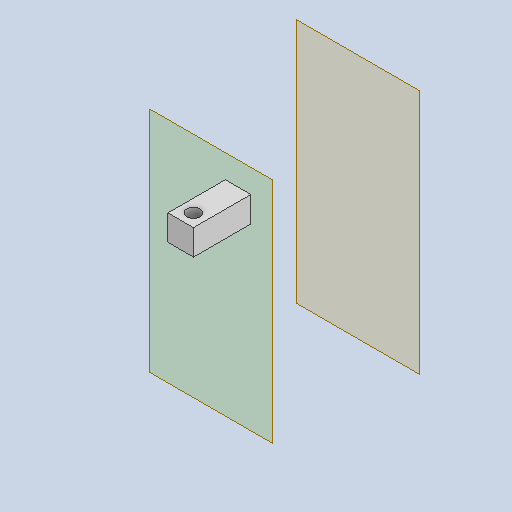
# Autodesk Inventor part: Refuerzo superior
Saved by Autodesk Inventor 2024 (Build 280153000, 153)
## iProperties
Created: 2025-03-01
Part Number: Refuerzo superior
Material: Genérico
Document SubType Name: Modeling
Designer: sergi
Density: 1 g/cm^3
Appearance: Valor por defecto
Author: sergi
Autodesk Inventor part; units mm, degrees
ref_plane "YZ Plane" through (0, 0, 0) normal (1, 0, 0) x (0, 1, 0)
ref_plane "XZ Plane" through (0, 0, 0) normal (0, 1, 0) x (-1, 0, 0)
sketch "Boceto1" plane through (0, 0, 0) normal (0, 1, 0) x (-1, 0, 0)
  line L0 (0, 0) -> (8, 0)
  line L1 (8, 0) -> (8, 66)
  line L2 (8, 66) -> (0, 66)
  line L3 (0, 66) -> (0, 0)
  dimension "d0" = 8
  dimension "d1" = 66
  constraints: 8 end point, 2 parallel, 1 horizontal, 1 perpendicular
  measures "d0" distance of L2.end L1.end
  measures "d1" distance of L1.end L0.end
extrude "Extrusión1" add sketch "Boceto1" along normal blind 8
ref_plane "Plano de trabajo1" through (-12.4, -21.9, 10) normal (0, 0, 1) x (1, 0, 0)
sketch "Boceto2" plane through (-12.4, -21.9, 10) normal (0, 0, 1) x (1, 0, 0)
  line L0 (4.4, 21.9) -> (12.4, 21.9) projected
  line L1 (12.4, 21.9) -> (12.4, 29.9) projected
  line L2 (4.4, 29.9) -> (12.4, 29.9) projected
  line L3 (4.4, 21.9) -> (4.4, 29.9) projected
  line L4 (3.4, 30.9) -> (13.4, 30.9)
  line L5 (13.4, 30.9) -> (13.4, 20.9)
  line L6 (13.4, 20.9) -> (3.4, 20.9)
  line L7 (3.4, 20.9) -> (3.4, 30.9)
  line L8 (4.4, 21.9) -> (3.4, 21.9)
  line L9 (12.4, 21.9) -> (13.4, 21.9)
  dimension "d23" = 1
  constraints: 12 end point, 3 point on line, 1 horizontal, 3 other
  measures "d23" distance between parallel lines of L3 L7
ref_plane "Plano de trabajo2" through (-29.9, -56.9, 56) normal (0, 0, -1) x (0, 1, 0)
extrude "Extrusión2" add sketch "Boceto2" along normal up to surface (46 mm away) contours L8 L7 L4 L5 L9 L1 L2 L3
sketch "Boceto3" plane through (-8, 0, 66) normal (0, 0, 1) x (1, 0, 0)
  line L0 (0, 0) -> (8, 0) projected
  line L1 (8, 0) -> (8, 8) projected
  line L2 (0, 8) -> (8, 8) projected
  line L3 (0, 0) -> (0, 8) projected
extrude "Extrusión3" add sketch "Boceto3" along normal blind 8
sketch "Boceto4" plane through (0, 0, 0) normal (0, 0, -1) x (-1, 0, 0)
  line L0 (0, 0) -> (8, 0) projected
  line L1 (8, 0) -> (8, 8) projected
  line L2 (0, 8) -> (8, 8) projected
  line L3 (0, 0) -> (0, 8) projected
extrude "Extrusión4" add sketch "Boceto4" along normal blind 8
sketch "Boceto5" plane through (0, 8, 0) normal (0, 1, 0) x (1, 0, 0)
  line L0 (-8, -10) -> (-8, 8) projected
  line L1 (0, -74) -> (-8, -74) projected
  line L2 (0, -56) -> (0, -74) projected
  line L3 (-8, 8) -> (0, 8) projected
  line L4 (0, 8) -> (-8, 8)
  line L5 (-8, 8) -> (-8, 0)
  line L6 (-8, 0) -> (0, 0)
  line L7 (0, 0) -> (0, 8)
  line L8 (0, -74) -> (-8, -74)
  line L9 (-8, -74) -> (-8, -66)
  line L10 (-8, -66) -> (0, -66)
  line L11 (0, -66) -> (0, -74)
  line L12 (0, 8) -> (-8, 0)
  line L13 (0, -74) -> (-8, -66)
  circle A0 centre (-4, 4) radius 2.1
  circle A1 centre (-4, -70) radius 2.1
  line L14 (-8, -10) -> (0, -10) projected
  line L15 (0, -10) -> (0, 8) projected
  line L16 (0, -56) -> (-8, -56) projected
  line L17 (-8, -56) -> (-8, -74) projected
  point P0 (0, 0)
  dimension "d11" = 4.2
  dimension "d12" = 4.2
  dimension "d13" = 8
  dimension "d14" = 8
  constraints: 20 end point, 4 parallel, 3 perpendicular, 2 centre point, 2 horizontal, 2 midpoint, 2 point on line
  measures "d11" diameter of A0
  measures "d12" diameter of A1
  measures "d13" distance between parallel lines of L3 L6
  measures "d14" distance between parallel lines of L10 L1
hole "Agujero1" at (-4, 8, -4) at (-4, 8, 70) direction (0, -1, 0) diameter 4.2 end through all
ref_plane "Plano de trabajo3" through (-12.4, -15.4, 56) normal (0, 0, -1) x (-1, 0, 0)
split "Dividir1" plane through (-12.4, -15.4, 56) removes the side toward (0, 0, -1)
